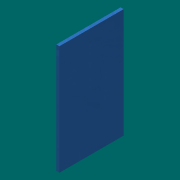
# Autodesk Inventor part: mirrorSides
Saved by Autodesk Inventor 2016 (Build 200138000, 138)
## iProperties
Created: 2015-10-14
Part Number: mirrorSides
Material: Glass
Document SubType Name: Modeling
Designer: Sawaiz
Density: 2.18 g/cm^3
Appearance: Cyan
Author: Sawaiz
Autodesk Inventor part; units mm, degrees
ref_plane "YZ Plane" through (0, 0, 0) normal (1, 0, 0) x (0, 1, 0)
ref_plane "XZ Plane" through (0, 0, 0) normal (0, 1, 0) x (-1, 0, 0)
ref_plane "XY Plane" through (0, 0, 0) normal (0, 0, 1) x (1, 0, 0)
sketch "Sketch1" plane through (0, 0, 0) normal (0, 1, 0) x (-1, 0, 0)
  line L0 (-40.7673, -53.175) -> (40.7673, -53.175)
  line L1 (40.7673, -53.175) -> (40.7673, 53.175)
  line L2 (40.7673, 53.175) -> (-40.7673, 53.175)
  line L3 (-40.7673, 53.175) -> (-40.7673, -53.175)
  line L4 (-40.7673, -53.175) -> (40.7673, 53.175) construction
  line L5 (40.7673, -53.175) -> (-40.7673, 53.175) construction
  point P0 (0, 0)
  dimension "d0" = 81.5345
  dimension "d1" = 106.35
  constraints: 12 end point, 2 midpoint, 2 parallel, 1 horizontal, 1 perpendicular
  measures "d0" distance of L2.end L1.end
  measures "d1" distance between parallel lines of L0 L2
extrude "Extrusion1" add sketch "Sketch1" along normal blind 3
equation "\"d1\" = height + acrylicThickness"
equation "\"d2\" = mirrorThickness"
equation "\"acrylicThickness\" = 6.35"
equation "\"height\" = 100"
equation "\"mirrorAngle\" = 16deg"
equation "\"detectorWidth\" = 52"
equation "\"detectorHeight\" = 52"
equation "\"mirrorThickness\" = 3"
equation "\"fresnelThickness\" = 0.1"
equation "\"focalLength\" = 76.2"
equation "\"ior\" = 1.49"
equation "\"centerThickness\" = 1.524"
equation "\"fresnelAngle\" = 90deg"
equation "\"fresnelEffectiveDiameter\" = 76.2"
body "Solid1"
